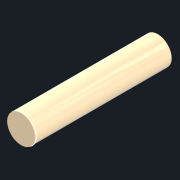
# Autodesk Inventor part: InteralBatHousing
Saved by Autodesk Inventor 2022.2 (Build 262287000, 287)
## iProperties
Created: 2022-01-31
Part Number: InteralBatHousing
Material: Polyethylene, Low Density
Document SubType Name: Modeling
Designer: Michael Lacey
Mass: 13.6111 g
Surface Area: 240.878 cm^2
Volume: 15.225 cm^3
Density: 0.894 g/cm^3
Appearance: Smooth - Off-White
Author: Michael Lacey
Autodesk Inventor part; units mm, degrees
ref_plane "YZ Plane" through (0, 0, 0) normal (1, 0, 0) x (0, 1, 0)
ref_plane "Work Plane1" through (-9.3053, -9.3053, -203.6437) normal (0, 0, -1) x (-0.6828, 0.7306, 0)
ref_plane "Work Plane2" through (-9.9277, -9.9277, -135.7625) normal (0, 0, -1) x (-0.6828, 0.7306, 0)
sketch "Sketch1" plane through (0, 0, 0) normal (0, 0, 1) x (1, 0, 0)
  circle A0 centre (0, 0) radius 12.7
  circle A1 centre (0, 0) radius 13.97
  dimension "d6" = 1.27
  dimension "d7" = 25.4
  constraints: 2 centre point, 2 coincident
  measures "d6" radial gap between concentric circles of A1 A0
  measures "d7" diameter of A0
extrude "Extrusion1" add sketch "Sketch1" against normal up to surface (135.7625 mm away)
sketch "Sketch2" plane through (0, 0, 0) normal (0, 0, 1) x (1, 0, 0)
  circle A0 centre (0, 0) radius 13.97 projected
extrude "Extrusion3" add sketch "Sketch2" along normal blind 1.27
body "Solid1"
